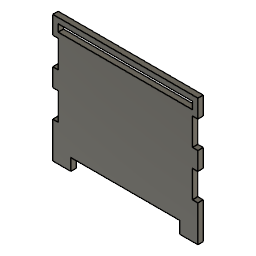
Muur Kort (Autodesk Fusion 360 design; units mm, degrees)
part number: 2026-03-12-09-15-02-357
Autodesk Fusion 360 part; units mm, degrees
sketch "Sketch1" plane through (0, 0, 0) normal (0, 0, 1) x (1, 0, 0)
  line L0 (-28.6561, 0.7869) -> (51.3439, 0.7869)
  line L1 (51.3439, 0.7869) -> (51.3439, -2.2131)
  line L2 (51.3439, -2.2131) -> (-28.6561, -2.2131)
  line L3 (-28.6561, -2.2131) -> (-28.6561, 0.7869)
  dimension "d1" = 3
  dimension "d2" = 80
  constraint horizontal L0
  constraint vertical L1
  constraint horizontal L2
  constraint vertical L3
  measures "d1" distance of L0.start L2.end
  measures "d2" distance of L1.end L2.end
extrude "Extrude1" add sketch "Sketch1" along normal blind 70
sketch "Sketch2" plane through (0, -2.2131, 0) normal (0, -1, 0) x (1, 0, 0)
  line L0 (-28.6561, 0) -> (51.3439, 0)
  line L1 (51.3439, 0) -> (51.3439, 70)
  line L2 (51.3439, 70) -> (-28.6561, 70)
  line L3 (-28.6561, 70) -> (-28.6561, 0)
  line L4 (-18.6561, 0) -> (41.3439, 0)
  line L5 (41.3439, 0) -> (41.3439, 6.61)
  line L6 (41.3439, 6.61) -> (-18.6561, 6.61)
  line L7 (-18.6561, 6.61) -> (-18.6561, 0)
  dimension "d5" = 10
  dimension "d6" = 60
  constraint horizontal L4
  constraint vertical L5
  constraint horizontal L6
  constraint vertical L7
  constraint coincident L0 L4.start
  measures "d5" distance of L0.start L4.start
  measures "d6" distance of L4.start L4.end
extrude "Extrude2" cut sketch "Sketch2" against normal blind 15 contours L0 L4 L5 L6 L7
sketch "Sketch3" plane through (0, -2.2131, 0) normal (0, -1, 0) x (1, 0, 0)
  line L0 (-18.6561, 0) -> (-18.6561, 6.61)
  line L1 (-18.6561, 6.61) -> (41.3439, 6.61)
  line L2 (41.3439, 6.61) -> (41.3439, 0)
  line L3 (41.3439, 0) -> (51.3439, 0)
  line L4 (51.3439, 0) -> (51.3439, 70)
  line L5 (51.3439, 70) -> (-28.6561, 70)
  line L6 (-28.6561, 70) -> (-28.6561, 0)
  line L7 (-28.6561, 0) -> (-18.6561, 0)
  line L8 (59.8727, 60) -> (-42.4062, 60) construction
  line L9 (-42.8479, 45) -> (61.1574, 45) construction
  line L10 (63.7389, 35) -> (-40.2664, 35) construction
  line L11 (-40.2664, 20) -> (63.7389, 20) construction
  line L12 (48.3439, -12.0113) -> (48.3439, -4.8877)
  line L13 (48.3439, -4.8877) -> (48.3439, 80.5961) construction
  line L14 (-25.6561, 80.5961) -> (-25.6561, -19.135) construction
  line L15 (-25.6561, 60) -> (-28.6561, 60)
  line L16 (-28.6561, 60) -> (-28.6561, 45)
  line L17 (-28.6561, 45) -> (-25.6561, 45)
  line L18 (-25.6561, 45) -> (-25.6561, 60)
  line L19 (-25.6561, 35) -> (-28.6561, 35)
  line L20 (-28.6561, 35) -> (-28.6561, 20)
  line L21 (-28.6561, 20) -> (-25.6561, 20)
  line L22 (-25.6561, 20) -> (-25.6561, 35)
  line L23 (48.3439, 20) -> (51.3439, 20)
  line L24 (51.3439, 20) -> (51.3439, 35)
  line L25 (51.3439, 35) -> (48.3439, 35)
  line L26 (48.3439, 35) -> (48.3439, 20)
  line L27 (48.3439, 45) -> (51.3439, 45)
  line L28 (51.3439, 45) -> (51.3439, 60)
  line L29 (51.3439, 60) -> (48.3439, 60)
  line L30 (48.3439, 60) -> (48.3439, 45)
  line L31 (-25.6561, 67) -> (48.3439, 67)
  line L32 (48.3439, 67) -> (48.3439, 63)
  line L33 (48.3439, 63) -> (-25.6561, 63)
  line L34 (-25.6561, 63) -> (-25.6561, 67)
  dimension "d9" = 3
  dimension "d10" = 3
  dimension "d11" = 10
  dimension "d12" = 15
  dimension "d13" = 10
  dimension "d14" = 15
  dimension "d17" = 4
  dimension "d18" = 3
  constraint perpendicular L6 L8
  constraint parallel L8 L9
  constraint perpendicular L6 L10
  constraint parallel L10 L11
  constraint perpendicular L11 L12
  constraint perpendicular L8 L13
  constraint perpendicular L1 L14
  constraint horizontal L15
  constraint vertical L16
  constraint horizontal L17
  constraint vertical L18
  constraint coincident L9 L16.end
  constraint coincident L6 L16.end
  constraint coincident L14 L15.start
  constraint coincident L8 L15.start
  constraint horizontal L19
  constraint vertical L20
  constraint horizontal L21
  constraint vertical L22
  constraint coincident L11 L20.end
  constraint coincident L6 L20.end
  constraint coincident L10 L19.start
  constraint coincident L14 L19.start
  constraint horizontal L23
  constraint vertical L24
  constraint horizontal L25
  constraint vertical L26
  constraint coincident L10 L24.end
  constraint coincident L4 L24.end
  constraint coincident L11 L23.start
  constraint coincident L13 L23.start
  constraint horizontal L27
  constraint vertical L28
  constraint horizontal L29
  constraint vertical L30
  constraint coincident L8 L28.end
  constraint coincident L4 L28.end
  constraint coincident L9 L27.start
  constraint coincident L13 L27.start
  constraint horizontal L31
  constraint vertical L32
  constraint horizontal L33
  constraint vertical L34
  constraint coincident L13 L32.end
  constraint coincident L14 L31.start
  measures "d9" distance of L6 L14
  measures "d10" distance of L4 L13
  measures "d11" distance of L5 L8
  measures "d12" distance of L8 L9
  measures "d13" distance of L9 L10
  measures "d14" distance of L10 L11
  measures "d17" distance of L31.end L32.end
  measures "d18" distance of L8 L33
extrude "Extrude3" cut sketch "Sketch3" against normal blind 10 contours L6 L19 L20 L21 L22 | L6 L15 L16 L17 L18 | L4 L23 L24 L25 L26 | L4 L27 L28 L29 L30 | L31 L32 L33 L34
